Autodesk Inventor part; units mm, degrees
(part 2 of 2)
sketch "Sketch7" plane through (-104.0575, 292.5377, -209.4) normal (0, 1, 0) x (1, 0, 0)
  line L0 (1.5076, 10.4067) -> (15.699, 10.4067) construction
  line L1 (15.699, 10.4067) -> (15.699, 0.6419) construction
  line L2 (15.699, 0.6419) -> (1.5076, 0.6419) construction
  line L3 (1.5076, 0.6419) -> (1.5076, 10.4067) construction
  spline S0 degree 2 poles (4.4589, 4.1928) (3.8755, 4.1928) (2.8884, 4.5866) (2.5286, 4.9804) knots 0 0 0 1 2 2 2
  spline S1 degree 2 poles (2.5286, 4.9804) (2.1688, 5.3694) (1.775, 6.5364) (1.775, 7.2949) knots 0 0 0 1 2 2 2
  spline S2 degree 2 poles (1.775, 7.2949) (1.775, 8.0485) (2.1591, 9.1668) (2.5238, 9.5801) knots 0 0 0 1 2 2 2
  spline S3 degree 2 poles (2.5238, 9.5801) (2.8836, 9.9837) (3.8657, 10.4067) (4.4735, 10.4067) knots 0 0 0 1 2 2 2
  spline S4 degree 2 poles (4.4735, 10.4067) (4.775, 10.4067) (5.305, 10.3192) (5.5286, 10.2511) knots 0 0 0 1 2 2 2
  spline S5 degree 2 poles (5.5286, 10.2511) (5.7231, 10.1879) (6.1267, 10.008) (6.326, 9.901) knots 0 0 0 1 2 2 2
  line L4 (6.326, 9.901) -> (6.326, 8.9383)
  line L5 (6.326, 8.9383) -> (6.2628, 8.9383)
  spline S6 degree 2 poles (6.2628, 8.9383) (6.1559, 9.0355) (5.8252, 9.3078) (5.587, 9.4391) knots 0 0 0 1 2 2 2
  spline S7 degree 2 poles (5.587, 9.4391) (5.3584, 9.5655) (4.8187, 9.726) (4.4687, 9.726) knots 0 0 0 1 2 2 2
  spline S8 degree 2 poles (4.4687, 9.726) (4.0845, 9.726) (3.399, 9.4099) (3.1413, 9.1085) knots 0 0 0 1 2 2 2
  spline S9 degree 2 poles (3.1413, 9.1085) (2.8884, 8.8022) (2.6064, 7.8735) (2.6064, 7.2949) knots 0 0 0 1 2 2 2
  spline S10 degree 2 poles (2.6064, 7.2949) (2.6064, 6.6774) (2.903, 5.7876) (3.1607, 5.4813) knots 0 0 0 1 2 2 2
  spline S11 degree 2 poles (3.1607, 5.4813) (3.4136, 5.1847) (4.0894, 4.8832) (4.4687, 4.8832) knots 0 0 0 1 2 2 2
  spline S12 degree 2 poles (4.4687, 4.8832) (4.8139, 4.8832) (5.4022, 5.0534) (5.6307, 5.1798) knots 0 0 0 1 2 2 2
  spline S13 degree 2 poles (5.6307, 5.1798) (5.8495, 5.3062) (6.1753, 5.5688) (6.2677, 5.6612) knots 0 0 0 1 2 2 2
  line L6 (6.2677, 5.6612) -> (6.326, 5.6612)
  line L7 (6.326, 5.6612) -> (6.326, 4.7082)
  spline S14 degree 2 poles (6.326, 4.7082) (6.1267, 4.6158) (5.7766, 4.4456) (5.5286, 4.3678) knots 0 0 0 1 2 2 2
  spline S15 degree 2 poles (5.5286, 4.3678) (5.2661, 4.2803) (4.8187, 4.1928) (4.4589, 4.1928) knots 0 0 0 1 2 2 2
  spline S16 degree 2 poles (9.5205, 4.7762) (9.4281, 4.7082) (9.117, 4.465) (8.9711, 4.3921) knots 0 0 0 1 2 2 2
  spline S17 degree 2 poles (8.9711, 4.3921) (8.7717, 4.2851) (8.3973, 4.1733) (8.057, 4.1733) knots 0 0 0 1 2 2 2
  spline S18 degree 2 poles (8.057, 4.1733) (7.7798, 4.1733) (7.279, 4.3824) (7.0894, 4.572) knots 0 0 0 1 2 2 2
  spline S19 degree 2 poles (7.0894, 4.572) (6.9095, 4.7568) (6.6907, 5.3014) (6.6907, 5.6028) knots 0 0 0 1 2 2 2
  spline S20 degree 2 poles (6.6907, 5.6028) (6.6907, 6.0696) (7.0845, 6.7308) (7.5124, 6.9205) knots 0 0 0 1 2 2 2
  spline S21 degree 2 poles (7.5124, 6.9205) (7.8917, 7.0955) (8.9225, 7.2268) (9.5205, 7.2608) knots 0 0 0 1 2 2 2
  line L8 (9.5205, 7.2608) -> (9.5205, 7.4067)
  spline S22 degree 2 poles (9.5205, 7.4067) (9.5205, 7.6693) (9.3601, 7.995) (9.2142, 8.0874) knots 0 0 0 1 2 2 2
  spline S23 degree 2 poles (9.2142, 8.0874) (9.0683, 8.1798) (8.6502, 8.2381) (8.4265, 8.2381) knots 0 0 0 1 2 2 2
  spline S24 degree 2 poles (8.4265, 8.2381) (8.164, 8.2381) (7.4541, 8.0825) (7.0991, 7.9318) knots 0 0 0 1 2 2 2
  line L9 (7.0991, 7.9318) -> (7.0554, 7.9318)
  line L10 (7.0554, 7.9318) -> (7.0554, 8.7049)
  spline S25 degree 2 poles (7.0554, 8.7049) (7.2644, 8.7633) (8.0473, 8.9091) (8.4314, 8.9091) knots 0 0 0 1 2 2 2
  spline S26 degree 2 poles (8.4314, 8.9091) (8.8982, 8.9091) (9.5351, 8.7633) (9.7879, 8.5736) knots 0 0 0 1 2 2 2
  spline S27 degree 2 poles (9.7879, 8.5736) (10.0359, 8.3889) (10.279, 7.8005) (10.279, 7.3775) knots 0 0 0 1 2 2 2
  line L11 (10.279, 7.3775) -> (10.279, 4.2997)
  line L12 (10.279, 4.2997) -> (9.5205, 4.2997)
  line L13 (9.5205, 4.2997) -> (9.5205, 4.7762)
  line L14 (9.5205, 5.4083) -> (9.5205, 6.6579)
  spline S28 degree 2 poles (9.5205, 6.6579) (9.2482, 6.6336) (8.4265, 6.5509) (8.1688, 6.4731) knots 0 0 0 1 2 2 2
  spline S29 degree 2 poles (8.1688, 6.4731) (7.8674, 6.3808) (7.4735, 5.9967) (7.4735, 5.6563) knots 0 0 0 1 2 2 2
  spline S30 degree 2 poles (7.4735, 5.6563) (7.4735, 5.2673) (7.9111, 4.8735) (8.3293, 4.8735) knots 0 0 0 1 2 2 2
  spline S31 degree 2 poles (8.3293, 4.8735) (8.6842, 4.8735) (9.2677, 5.1798) (9.5205, 5.4083) knots 0 0 0 1 2 2 2
  line L15 (16.4492, 4.2997) -> (16.4492, 6.9059)
  spline S32 degree 2 poles (16.4492, 6.9059) (16.4492, 7.2171) (16.4006, 7.7471) (16.3228, 7.8929) knots 0 0 0 1 2 2 2
  spline S33 degree 2 poles (16.3228, 7.8929) (16.245, 8.0534) (15.9484, 8.209) (15.6907, 8.209) knots 0 0 0 1 2 2 2
  spline S34 degree 2 poles (15.6907, 8.209) (15.4573, 8.209) (14.9225, 7.9221) (14.6405, 7.6498) knots 0 0 0 1 2 2 2
  spline S35 degree 2 poles (14.6405, 7.6498) (14.6453, 7.5817) (14.655, 7.3921) (14.655, 7.2657) knots 0 0 0 1 2 2 2
  line L16 (14.655, 7.2657) -> (14.655, 4.2997)
  line L17 (14.655, 4.2997) -> (13.8965, 4.2997)
  line L18 (13.8965, 4.2997) -> (13.8965, 6.9059)
  spline S36 degree 2 poles (13.8965, 6.9059) (13.8965, 7.2171) (13.8479, 7.7471) (13.7701, 7.8929) knots 0 0 0 1 2 2 2
  spline S37 degree 2 poles (13.7701, 7.8929) (13.6923, 8.0534) (13.3957, 8.209) (13.138, 8.209) knots 0 0 0 1 2 2 2
  spline S38 degree 2 poles (13.138, 8.209) (12.8949, 8.209) (12.3552, 7.9026) (12.1024, 7.6644) knots 0 0 0 1 2 2 2
  line L19 (12.1024, 7.6644) -> (12.1024, 4.2997)
  line L20 (12.1024, 4.2997) -> (11.3439, 4.2997)
  line L21 (11.3439, 4.2997) -> (11.3439, 8.8022)
  line L22 (11.3439, 8.8022) -> (12.1024, 8.8022)
  line L23 (12.1024, 8.8022) -> (12.1024, 8.3062)
  spline S39 degree 2 poles (12.1024, 8.3062) (12.399, 8.6028) (12.9824, 8.9286) (13.3325, 8.9286) knots 0 0 0 1 2 2 2
  spline S40 degree 2 poles (13.3325, 8.9286) (13.7312, 8.9286) (14.3487, 8.5639) (14.5092, 8.1506) knots 0 0 0 1 2 2 2
  spline S41 degree 2 poles (14.5092, 8.1506) (14.8544, 8.5347) (15.5059, 8.9286) (15.8852, 8.9286) knots 0 0 0 1 2 2 2
  spline S42 degree 2 poles (15.8852, 8.9286) (16.1769, 8.9286) (16.6534, 8.7487) (16.8285, 8.5445) knots 0 0 0 1 2 2 2
  spline S43 degree 2 poles (16.8285, 8.5445) (17.0084, 8.3402) (17.2077, 7.7276) (17.2077, 7.2657) knots 0 0 0 1 2 2 2
  line L24 (17.2077, 7.2657) -> (17.2077, 4.2997)
  line L25 (17.2077, 4.2997) -> (16.4492, 4.2997)
  spline S44 degree 2 poles (20.2272, 4.1976) (19.1478, 4.1976) (17.9614, 5.4083) (17.9614, 6.5266) knots 0 0 0 1 2 2 2
  spline S45 degree 2 poles (17.9614, 6.5266) (17.9614, 7.6255) (19.1137, 8.9286) (20.0424, 8.9286) knots 0 0 0 1 2 2 2
  spline S46 degree 2 poles (20.0424, 8.9286) (20.4606, 8.9286) (21.1072, 8.6855) (21.3455, 8.4278) knots 0 0 0 1 2 2 2
  spline S47 degree 2 poles (21.3455, 8.4278) (21.5886, 8.1701) (21.8463, 7.4261) (21.8463, 6.8864) knots 0 0 0 1 2 2 2
  line L26 (21.8463, 6.8864) -> (21.8463, 6.4731)
  line L27 (21.8463, 6.4731) -> (18.7296, 6.4731)
  spline S48 degree 2 poles (18.7296, 6.4731) (18.7296, 5.6903) (19.5173, 4.8589) (20.2174, 4.8589) knots 0 0 0 1 2 2 2
  spline S49 degree 2 poles (20.2174, 4.8589) (20.4654, 4.8589) (20.9468, 4.9707) (21.1413, 5.0582) knots 0 0 0 1 2 2 2
  spline S50 degree 2 poles (21.1413, 5.0582) (21.3455, 5.1555) (21.6275, 5.3257) (21.7199, 5.4035) knots 0 0 0 1 2 2 2
  line L28 (21.7199, 5.4035) -> (21.7636, 5.4035)
  line L29 (21.7636, 5.4035) -> (21.7636, 4.5769)
  spline S51 degree 2 poles (21.7636, 4.5769) (21.6324, 4.5234) (21.2337, 4.3678) (21.0781, 4.324) knots 0 0 0 1 2 2 2
  spline S52 degree 2 poles (21.0781, 4.324) (20.8593, 4.2608) (20.4995, 4.1976) (20.2272, 4.1976) knots 0 0 0 1 2 2 2
  spline S53 degree 2 poles (21.1072, 7.0518) (21.0975, 7.3581) (20.9711, 7.8054) (20.8495, 7.9561) knots 0 0 0 1 2 2 2
  spline S54 degree 2 poles (20.8495, 7.9561) (20.7183, 8.1263) (20.305, 8.3062) (19.9986, 8.3062) knots 0 0 0 1 2 2 2
  spline S55 degree 2 poles (19.9986, 8.3062) (19.6972, 8.3062) (19.2742, 8.1263) (19.0991, 7.9513) knots 0 0 0 1 2 2 2
  spline S56 degree 2 poles (19.0991, 7.9513) (18.929, 7.7714) (18.7539, 7.3386) (18.7296, 7.0518) knots 0 0 0 1 2 2 2
  line L30 (18.7296, 7.0518) -> (21.1072, 7.0518)
  line L31 (25.0019, 7.9902) -> (24.963, 7.9902)
  spline S57 degree 2 poles (24.963, 7.9902) (24.8755, 8.0145) (24.6858, 8.0242) (24.5546, 8.0242) knots 0 0 0 1 2 2 2
  spline S58 degree 2 poles (24.5546, 8.0242) (24.2482, 8.0242) (23.6453, 7.7568) (23.373, 7.4942) knots 0 0 0 1 2 2 2
  line L32 (23.373, 7.4942) -> (23.373, 4.2997)
  line L33 (23.373, 4.2997) -> (22.6145, 4.2997)
  line L34 (22.6145, 4.2997) -> (22.6145, 8.8022)
  line L35 (22.6145, 8.8022) -> (23.373, 8.8022)
  line L36 (23.373, 8.8022) -> (23.373, 8.1312)
  spline S59 degree 2 poles (23.373, 8.1312) (23.7863, 8.5007) (24.4038, 8.8022) (24.6956, 8.8022) knots 0 0 0 1 2 2 2
  spline S60 degree 2 poles (24.6956, 8.8022) (24.8123, 8.8022) (24.929, 8.7924) (25.0019, 8.7778) knots 0 0 0 1 2 2 2
  line L37 (25.0019, 8.7778) -> (25.0019, 7.9902)
  spline S61 degree 2 poles (28.0991, 4.7762) (28.0067, 4.7082) (27.6956, 4.465) (27.5497, 4.3921) knots 0 0 0 1 2 2 2
  spline S62 degree 2 poles (27.5497, 4.3921) (27.3503, 4.2851) (26.976, 4.1733) (26.6356, 4.1733) knots 0 0 0 1 2 2 2
  spline S63 degree 2 poles (26.6356, 4.1733) (26.3584, 4.1733) (25.8576, 4.3824) (25.668, 4.572) knots 0 0 0 1 2 2 2
  spline S64 degree 2 poles (25.668, 4.572) (25.4881, 4.7568) (25.2693, 5.3014) (25.2693, 5.6028) knots 0 0 0 1 2 2 2
  spline S65 degree 2 poles (25.2693, 5.6028) (25.2693, 6.0696) (25.6631, 6.7308) (26.091, 6.9205) knots 0 0 0 1 2 2 2
  spline S66 degree 2 poles (26.091, 6.9205) (26.4703, 7.0955) (27.5011, 7.2268) (28.0991, 7.2608) knots 0 0 0 1 2 2 2
  line L38 (28.0991, 7.2608) -> (28.0991, 7.4067)
  spline S67 degree 2 poles (28.0991, 7.4067) (28.0991, 7.6693) (27.9387, 7.995) (27.7928, 8.0874) knots 0 0 0 1 2 2 2
  spline S68 degree 2 poles (27.7928, 8.0874) (27.6469, 8.1798) (27.2288, 8.2381) (27.0051, 8.2381) knots 0 0 0 1 2 2 2
  spline S69 degree 2 poles (27.0051, 8.2381) (26.7426, 8.2381) (26.0327, 8.0825) (25.6777, 7.9318) knots 0 0 0 1 2 2 2
  line L39 (25.6777, 7.9318) -> (25.634, 7.9318)
  line L40 (25.634, 7.9318) -> (25.634, 8.7049)
  spline S70 degree 2 poles (25.634, 8.7049) (25.8431, 8.7633) (26.6259, 8.9091) (27.01, 8.9091) knots 0 0 0 1 2 2 2
  spline S71 degree 2 poles (27.01, 8.9091) (27.4768, 8.9091) (28.1137, 8.7633) (28.3666, 8.5736) knots 0 0 0 1 2 2 2
  spline S72 degree 2 poles (28.3666, 8.5736) (28.6145, 8.3889) (28.8576, 7.8005) (28.8576, 7.3775) knots 0 0 0 1 2 2 2
  line L41 (28.8576, 7.3775) -> (28.8576, 4.2997)
  line L42 (28.8576, 4.2997) -> (28.0991, 4.2997)
  line L43 (28.0991, 4.2997) -> (28.0991, 4.7762)
  line L44 (28.0991, 5.4083) -> (28.0991, 6.6579)
  spline S73 degree 2 poles (28.0991, 6.6579) (27.8268, 6.6336) (27.0051, 6.5509) (26.7474, 6.4731) knots 0 0 0 1 2 2 2
  spline S74 degree 2 poles (26.7474, 6.4731) (26.446, 6.3808) (26.0521, 5.9967) (26.0521, 5.6563) knots 0 0 0 1 2 2 2
  spline S75 degree 2 poles (26.0521, 5.6563) (26.0521, 5.2673) (26.4897, 4.8735) (26.9079, 4.8735) knots 0 0 0 1 2 2 2
  spline S76 degree 2 poles (26.9079, 4.8735) (27.2628, 4.8735) (27.8463, 5.1798) (28.0991, 5.4083) knots 0 0 0 1 2 2 2
  point P0 (104.0575, -209.4)
  dimension "d0" = 44
  dimension "d1" = 120
  dimension "d4" = 20
  dimension "d5" = 10
  constraints: 2 other
extrude "Extrusion11" add sketch "Sketch7" along normal blind 1
equation "\"d5\" = 0.5 * d4"
body "Solid1"
